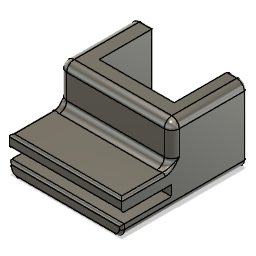
Thrust tester mount on glass v1 (Autodesk Fusion 360 design; units mm, degrees)
Autodesk Fusion 360 part; units mm, degrees
sketch "Sketch1" plane through (0, 0, 0) normal (0, 1, 0) x (1, 0, 0)
  line L0 (0, 0) -> (30, 0)
  line L1 (30, 0) -> (37, 0)
  line L2 (0, 0) -> (-8, 0)
  line L3 (-8, 0) -> (-8, -30)
  line L4 (0, 0) -> (0, -22)
  line L5 (30, 0) -> (30, -22)
  line L6 (37, 0) -> (37, -30)
  line L7 (30, -22) -> (0, -22)
  line L8 (37, -30) -> (-8, -30)
  dimension "d1" = 30
  dimension "d2" = 7
  dimension "d3" = 8
  dimension "d4" = 30
  dimension "d5" = 22
  constraint coincident L0.start L2.start
  constraint horizontal L0
  constraint parallel L0 L1
  constraint parallel L0 L2
  constraint perpendicular L2 L3
  constraint perpendicular L0 L4
  constraint perpendicular L0 L5
  constraint perpendicular L1 L6
  constraint perpendicular L4 L7
  constraint perpendicular L3 L8
  measures "d1" distance of L0.start L0.end
  measures "d2" distance of L0.end L1.end
  measures "d3" distance of L0.start L2.end
  measures "d4" distance of L2.end L3.end
  measures "d5" distance of L0.start L4.end L2.start
extrude "Extrude1" add sketch "Sketch1" along normal blind 30 contours L1 L2 L3 L4 L5 L6 L7 L8
sketch "Sketch2" plane through (-8, 0, 0) normal (-1, 0, 0) x (0, 0, 1)
  line L0 (0, 0) -> (30, 0)
  line L1 (30, 0) -> (30, 30)
  line L2 (30, 30) -> (0, 30)
  line L3 (0, 30) -> (0, 0)
  line L4 (30, 0) -> (50, 0)
  line L5 (50, 0) -> (50, 5)
  line L6 (50, 5) -> (30, 5)
  line L7 (30, 5) -> (30, 9.2)
  line L8 (30, 9.2) -> (50, 9.2)
  line L9 (50, 9.2) -> (50, 14.2)
  line L10 (50, 14.2) -> (47, 14.2)
  line L11 (47, 14.2) -> (30, 14.2)
  dimension "d8" = 20
  dimension "d9" = 5
  dimension "d10" = 4.2
  dimension "d11" = 5
  constraint coincident L0.end L1.start
  constraint perpendicular L1 L4
  constraint perpendicular L4 L5
  constraint coincident L1 L6.end
  constraint perpendicular L1 L6
  constraint perpendicular L6 L7
  constraint perpendicular L5 L8
  constraint perpendicular L8 L9
  constraint perpendicular L9 L10
  constraint coincident L1 L11.end
  constraint perpendicular L1 L11
  measures "d8" distance of L0.end L4.end
  measures "d9" distance of L4.end L5.end
  measures "d10" distance of L6.end L7.end
  measures "d11" distance of L8.end L9.end
extrude "Extrude2" add sketch "Sketch2" against normal up to surface (45 mm away) contours L1 L4 L5 L6 | L1 L8 L9 L10 L11
fillet "Fillet1" radius 3 8 edges at (14.5, 14.2, 30) (-8, 22.1, 30) (37, 22.1, 30) (37, 30, 15) (-8, 30, 15) (-8, 0, 25) (37, 0, 25) (14.5, 30, 30)
fillet "Fillet2" radius 1 12 edges at (14.5, 5, 50) (14.5, 9.2, 50) (14.5, 14.2, 50) (-8, 14.2, 41.0981) (-8, 15.157, 29.3391) (37, 14.2, 41.0981) (37, 15.157, 29.3391) (-8, 4, 50) (-7.1213, 0.8787, 50) (14.5, 0, 50) (36.1213, 0.8787, 50) (37, 4, 50)
fillet "Fillet3" radius 1 12 edges at (-2.5, 0, 0) (-7.1213, 0.8787, 0) (-8, 15, 0) (-7.1213, 29.1213, 0) (-2.5, 30, 0) (0, 15, 0) (30, 15, 0) (32, 0, 0) (36.1213, 0.8787, 0) (37, 15, 0) (36.1213, 29.1213, 0) (32, 30, 0)
